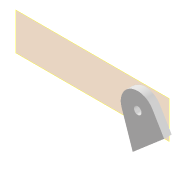
# Autodesk Inventor part: zijkant
Saved by Autodesk Inventor 2020.3 (Build 243373000, 373)
## iProperties
Created: 2020-09-15
Part Number: zijkant
Material: Generic
Document SubType Name: Modeling
Designer: Svend
Density: 1 g/cm^3
Appearance: Default
Author: Svend
Autodesk Inventor part; units mm, degrees
ref_plane "YZ Plane" through (0, 0, 0) normal (1, 0, 0) x (0, 1, 0)
ref_plane "XZ Plane" through (0, 0, 0) normal (0, 1, 0) x (-1, 0, 0)
ref_plane "XY Plane" through (0, 0, 0) normal (0, 0, 1) x (1, 0, 0)
ref_plane "Work Plane1" through (0, 0, 0) normal (0, 0, 1) x (1, 0, 0)
sketch "Sketch1" plane through (0, 0, 0) normal (0, 0, 1) x (1, 0, 0)
  circle A0 centre (70, 0) radius 5 projected
  circle A1 centre (293.8763, -377.7839) radius 4.188 projected
  circle A2 centre (293.8763, -377.7839) radius 8.8 projected
  arc A3 (63.7, -21.6) -> (-63.7, -21.6) centre (0, -240) ccw projected
  arc A4 (63.7, -21.6) -> (63.7, 21.6) centre (70, 0) ccw projected
  arc A5 (-63.7, 21.6) -> (63.7, 21.6) centre (0, 240) ccw projected
  arc A6 (-63.7, 21.6) -> (-63.7, -21.6) centre (-70, 0) ccw projected
  circle A7 centre (70, 0) radius 5 projected
  circle A8 centre (-70, 0) radius 5 projected
  arc A9 (103.2014, -50.6129) -> (104.1376, -47.9439) centre (102.335, -48.8103) ccw projected
  line L0 (104.1376, -47.9439) -> (88.9974, -16.4423) projected
  arc A10 (89.2305, -11.6806) -> (88.9974, -16.4423) centre (93.504, -14.2763) ccw projected
  arc A11 (89.2305, -11.6806) -> (67.1075, -22.3133) centre (70, 0) ccw projected
  arc A12 (70.9713, -25.1059) -> (67.1075, -22.3133) centre (66.4648, -27.2718) ccw projected
  line L1 (70.9713, -25.1059) -> (86.1115, -56.6076) projected
  arc A13 (86.1115, -56.6076) -> (88.7805, -57.5438) centre (87.9141, -55.7412) ccw projected
  line L2 (88.7805, -57.5438) -> (103.2014, -50.6129) projected
  circle A14 centre (70, 0) radius 5 projected
  circle A15 centre (90.3596, -42.3614) radius 3 projected
  line L3 (48.6704, -7.1624) -> (63.3384, -50.8434)
  line L4 (63.3384, -50.8434) -> (105.0547, -15)
  line L5 (105.0547, -15) -> (89.3527, 11.477)
  point P0 (0, 0)
  point P1 (89.3527, 11.477)
  dimension "d0" = 15
  dimension "d1" = 5
  dimension "d2" = 55
  dimension "d3" = 15
  constraints: 6 end point, 2 point on circle, 2 tangent
  measures "d0" angle of L4 L2
  measures "d1" angle of L0 L5
  measures "d2" distance of L3.end L4.end
  measures "d3" vertical distance of L4.end A0.centre
extrude "Extrusion1" add sketch "Sketch1" along normal blind 10 contours A4 A12 L1 L4 L3 A3 | A11 A4 | A3 L3 A11 | A4 A10 L0 L4 L1 A12 | A4 L5 L4 L0 A10
body "Solid1"
